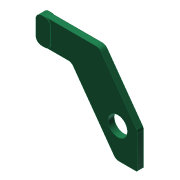
# Autodesk Inventor part: J002856
Saved by Autodesk Inventor 2012 SP2 (Build 160219200, 219)
## iProperties
Created: 2014-08-19
Material: STAINLESS STEEL, 303
Vendor: HHMI: JFRC - ID&F
Document SubType Name: Modeling
Designer: arnoldj
Density: 8 g/cm^3
Mass: 2.42747 g
Surface Area: 5.11631 cm^2
Volume: 0.303433 cm^3
Part Number: J002856
Description: MPS H Bar Clamp Top
Project: P-194005
RuleStatus: InUse
AfterDocSave0: file://Part Number Cleaner
LAB/DEPT: SVOBODA (LAB)
REQUESTING SCIENTIST: PERON, SIMON
SURFACE ROUGHNESS: 63 Ra
DESIGN DEPARTMENT: HHMI: JFRC - ID&F
SPECIAL FINISH: NONE
ALTERED ITEM PART NUMBER: N/A
ALTERED ITEM VENDOR: N/A
ALTERED ITEM DESCRIPTION: N/A
Revision Number: -
Autodesk Inventor part; units mm, degrees
ref_plane "YZ Plane" through (0, 0, 0) normal (1, 0, 0) x (0, 1, 0)
ref_plane "XZ Plane" through (0, 0, 0) normal (0, 1, 0) x (-1, 0, 0)
ref_plane "XY Plane" through (0, 0, 0) normal (0, 0, 1) x (1, 0, 0)
sketch "Sketch1" plane through (0, 0, 0) normal (0, 0, 1) x (1, 0, 0)
  line L0 (0, 0) -> (-4.699, 0)
  line L1 (-4.699, 0) -> (-14.3764, 13.4874)
  line L2 (-14.3764, 13.4874) -> (-21.9964, 13.4874)
  line L3 (-21.9964, 13.4874) -> (-21.9964, 19.2024)
  line L4 (-21.9964, 19.2024) -> (-8.3105, 19.2024)
  line L5 (-8.3105, 19.2024) -> (0, 7.62)
  line L6 (0, 7.62) -> (0, 0)
  line L7 (0, 23.0429) -> (0, -3.8405) projected
  line L8 (-26.3957, 0) -> (4.3993, 0) projected
  dimension "d0" = 7.62
  dimension "d1" = 5.715
  dimension "d2" = 4.699
  dimension "d3" = 19.2024
  dimension "d4" = 21.9964
  dimension "d5" = 7.62
  dimension "d6" = 13.6859
  dimension "d7" = 14.2554
  constraints: 14 end point, 4 parallel, 1 horizontal, 1 perpendicular
  measures "d0" distance of L5.end L0.start
  measures "d1" distance of L2.end L3.end
  measures "d2" distance of L0.start L0.end
  measures "d3" distance between parallel lines of L8 L4
  measures "d4" distance between parallel lines of L7 L3
  measures "d5" distance of L1.end L2.end
  measures "d6" distance of L3.end L4.end
  measures "d7" distance of L4.end L5.end
extrude "Extrusion1" add sketch "Sketch1" along normal blind 1.5875
sketch "Sketch2" plane through (0, 0, 0) normal (0, 0, 1) x (1, 0, 0)
  circle A0 centre (-4.2926, 6.5024) radius 0.635
  line L0 (-26.3957, 0) -> (4.3993, 0) projected
  line L1 (0, 23.0429) -> (0, -3.8405) projected
  line L2 (-21.9964, 13.4874) -> (-21.9964, 19.2024) projected
  line L3 (-21.9964, 19.2024) -> (-8.3105, 19.2024) projected
  point P0 (0, 0)
  dimension "d11" = 17.7038
  dimension "d12" = 12.7
  dimension "d13" = 1.27
  constraints: 1 centre point, 1 coincident
  measures "d11" distance from line of A0.centre L2
  measures "d12" distance from line of A0.centre L3
  measures "d13" diameter of A0
hole "Hole1" at (-4.2926, 6.5024, 0) direction (0, 0, 1) diameter 4.2164 end through all
fillet "Fillet1" radius 1.27 6 edges at (-21.9964, 13.4874, 0.7937) (-14.3764, 13.4874, 0.7937) (-4.699, 0, 0.7937) (0, 7.62, 0.7937) (-8.3105, 19.2024, 0.7937) (-21.9964, 19.2024, 0.7937)
fillet "Fillet2" radius 0.254 1 edges at (0, 0, 0.7937)
sketch "Sketch3" plane through (0, 0, 1.5875) normal (0, 0, 1) x (1, 0, 0)
  line L0 (-20.7264, 19.2024) -> (-8.9624, 19.2024) projected
  circle A0 centre (-4.2926, 6.5024) radius 2.1082 projected
  line L1 (0, 0) -> (-18.8214, 0)
  line L2 (-18.8214, 0) -> (-18.8214, 19.2024)
  line L3 (-18.8214, 19.2024) -> (0, 19.2024)
  line L4 (0, 19.2024) -> (0, 0)
  point P0 (-21.9964, 17.9324)
  dimension "d23" = 3.175
  constraints: 8 end point, 2 parallel, 1 horizontal, 1 perpendicular, 1 point on line
  measures "d23" distance from line of L2 point (-21.996, 17.932)
extrude "Extrusion2" cut sketch "Sketch3" against normal blind 0.127
sketch "Sketch4" plane through (0, 0, 0) normal (0, 0, -1) x (-1, 0, 0)
  circle A0 centre (4.2926, 6.5024) radius 2.1082 projected
  line L0 (21.9964, 14.7574) -> (21.9964, 17.9324) projected
  line L1 (20.7264, 19.2024) -> (8.9624, 19.2024) projected
  line L2 (0, 0) -> (18.8214, 0)
  line L3 (18.8214, 0) -> (18.8214, 19.2024)
  line L4 (18.8214, 19.2024) -> (0, 19.2024)
  line L5 (0, 19.2024) -> (0, 0)
  dimension "d26" = 3.175
  constraints: 8 end point, 2 parallel, 1 horizontal, 1 perpendicular, 1 point on line
  measures "d26" distance between parallel lines of L3 L0
extrude "Extrusion3" cut sketch "Sketch4" against normal blind 0.127
fillet "Fillet3" radius 1.27 4 edges at (-18.8214, 13.4874, 0.0635) (-18.8214, 19.2024, 0.0635) (-18.8214, 19.2024, 1.524) (-18.8214, 13.4874, 1.524)
body "Solid1"
